Display PCB Holder (Autodesk Fusion 360 design; units mm, degrees)
Autodesk Fusion 360 part; units mm, degrees
sketch "Sketch1" plane through (0, 0, 0) normal (0, 0, 1) x (1, 0, 0)
  line L0 (-91, 0) -> (-91, 66)
  line L1 (0, 66) -> (0, 0)
  line L2 (2, 68) -> (2, -2)
  line L3 (2, -2) -> (-93, -2)
  line L4 (-93, -2) -> (-93, 68)
  line L5 (-93, 68) -> (2, 68)
  line L6 (-89, 68) -> (-89, 66)
  line L7 (-2, 68) -> (-2, 66)
  line L8 (-89, 0) -> (-89, -2)
  line L9 (-2, 0) -> (-2, -2)
  line L10 (-91, 66) -> (-89, 66)
  line L11 (-2, 66) -> (0, 66)
  line L12 (0, 0) -> (-2, 0)
  line L13 (-89, 0) -> (-91, 0)
  dimension "d1" = 91
  dimension "d2" = 66
  dimension "d4" = 2
  dimension "d5" = 2
  dimension "d6" = 2
  dimension "d7" = 2
  constraint horizontal L12
  constraint vertical L0
  constraint horizontal L10
  constraint vertical L1
  constraint coincident L1.end L12.start
  constraint coincident L5 L6.start
  constraint perpendicular L6 L10
  constraint coincident L5 L7.start
  constraint coincident L7.end L10
  constraint perpendicular L7 L10
  constraint coincident L8.start L12
  constraint coincident L3 L8.end
  constraint perpendicular L3 L8
  constraint coincident L3 L9.end
  constraint perpendicular L3 L9
  constraint collinear L10 L11
  constraint parallel L1 L2
  constraint parallel L3 L12
  constraint parallel L0 L4
  constraint collinear L12 L13
  measures "d1" distance of L1.end L0.start
  measures "d2" distance of L1.end L1.start
  measures "d4" distance of L0.end L6
  measures "d5" distance of L1.start L7
  measures "d6" distance of L1.end L9
  measures "d7" distance of L0.start L8
extrude "Extrude2" add sketch "Sketch1" along normal blind 6 contours L0 L3 L4 L5 L6 L8 L10 L13 | L1 L2 L3 L5 L7 L9 L11 L12 makes body 1 at (-93, 21.3333, 2) makes body 2 at (2, 44.6667, 2)
extrude "Extrude1" add sketch "Sketch1" along normal blind 2 separate body contours L0 L1 L3 L5 L6 L7 L8 L9 L10 L11 L12 L13 makes body 3
